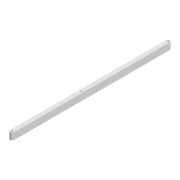
# Autodesk Inventor part: Part_5
Saved by Autodesk Inventor 2022 (Build 260153000, 153)
## iProperties
Created: 2022-05-03
Part Number: Part_5
Material: Generic
Document SubType Name: Modeling
Designer: dell
Density: 1 g/cm^3
Appearance: Default
Author: dell
Autodesk Inventor part; units mm, degrees
ref_plane "YZ Plane" through (0, 0, 0) normal (1, 0, 0) x (0, 1, 0)
ref_plane "XZ Plane" through (0, 0, 0) normal (0, 1, 0) x (-1, 0, 0)
ref_plane "XY Plane" through (0, 0, 0) normal (0, 0, 1) x (1, 0, 0)
sketch "Sketch1" plane through (0, 0, 0) normal (0, 1, 0) x (-1, 0, 0)
  line L0 (0, 0) -> (0, -233.234) construction
  line L1 (-3, 0) -> (-3, -233.234)
  line L2 (3, -233.234) -> (3, 0)
  arc A0 (3, 0) -> (-3, 0) centre (0, 0) ccw
  arc A1 (-3, -233.234) -> (3, -233.234) centre (0, -233.234) ccw
  circle A2 centre (0, 0) radius 1.5
  circle A3 centre (0, -233.234) radius 1.5
  circle A4 centre (0, -103.234) radius 1.5
  point P0 (0, -116.617)
  dimension "d0" = 6
  dimension "d1" = 233.234
  dimension "d2" = 3
  dimension "d3" = 3
  dimension "d16" = 3
  dimension "d17" = 103.234
  constraints: 8 end point, 5 centre point, 4 point on circle, 4 tangent, 2 coincident, 1 midpoint, 1 parallel, 1 point on line, 1 vertical
  measures "d0" diameter of A1
  measures "d1" distance of L0.end L0.start
  measures "d2" diameter of A2
  measures "d3" diameter of A3
  measures "d16" diameter of A4
  measures "d17" distance of L0.start A4.centre
extrude "Extrusion1" add sketch "Sketch1" along normal blind 10
body "Solid1"
